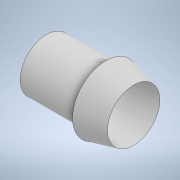
# Autodesk Inventor part: корпус фары
Saved by Autodesk Inventor 2021.2 (Build 252289000, 289)
## iProperties
Created: 2022-07-09
Part Number: корпус фары
Material: Типовые
Document SubType Name: Modeling
Designer: ROOT
Density: 1 g/cm^3
Appearance: По умолчанию
Author: ROOT
Autodesk Inventor part; units mm, degrees
ref_plane "YZ Plane" through (0, 0, 0) normal (1, 0, 0) x (0, 1, 0)
ref_plane "XZ Plane" through (0, 0, 0) normal (0, 1, 0) x (-1, 0, 0)
ref_plane "XY Plane" through (0, 0, 0) normal (0, 0, 1) x (1, 0, 0)
sketch "Эскиз1" plane through (0, 0, 0) normal (0, 0, 1) x (1, 0, 0)
  line L0 (0, 0) -> (-21.4884, 0)
  line L1 (0, 3.75) -> (-4, 4.75)
  line L2 (-4, 4.75) -> (-4, 3.75)
  line L3 (-4, 3.75) -> (-12.5, 3.75)
  line L4 (-12.5, 3.75) -> (-12.5, 3.25)
  line L5 (-12.5, 3.25) -> (-6, 3.25)
  line L6 (-6, 3.25) -> (-6, 2.75)
  line L7 (-6, 2.75) -> (0, 3.75)
  dimension "d1" = 8.5
  dimension "d2" = 1
  dimension "d3" = 0.5
  dimension "d4" = 6.5
  dimension "d5" = 4
  dimension "d6" = 0
  dimension "d9" = 3.75
  dimension "d10" = 2.75
  dimension "d11" = 3.75
  constraints: 16 end point, 3 perpendicular, 2 vertical, 1 horizontal
  measures "d1" distance of L2.end L3.end
  measures "d2" distance of L1.end L2.end
  measures "d3" distance of L3.end L4.end
  measures "d4" distance of L4.end L5.end
  measures "d5" horizontal distance of L1.start L1.end
  measures "d6" horizontal distance of L0.start L1.start
  measures "d9" distance of L0.start L1.start
  measures "d10" vertical distance of L0.start L6.end
  measures "d11" vertical distance of L0.start L3.end
revolve "Вращение1" add sketch "Эскиз1" angle 360 about axis through (0, 0, 0) along (-1, 0, 0)
